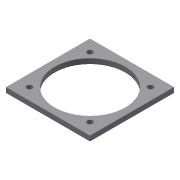
# Autodesk Inventor part: chamberPlateNA11_thin
Saved by Autodesk Inventor 2013 (Build 170138000, 138)
## iProperties
Created: 2012-12-03
Part Number: chamberPlateNA11_thin
Document SubType Name: Modeling
Designer: Ke Si
Density: 1 g/cm^3
Material: Generic
Author: Ke Si
Autodesk Inventor part; units mm, degrees
ref_plane "YZ Plane" through (0, 0, 0) normal (1, 0, 0) x (0, 1, 0)
ref_plane "XZ Plane" through (0, 0, 0) normal (0, 1, 0) x (-1, 0, 0)
ref_plane "XY Plane" through (0, 0, 0) normal (0, 0, 1) x (1, 0, 0)
sketch "Sketch7" plane through (0, 0, 0) normal (0, 1, 0) x (-1, 0, 0)
  line L0 (-25, -25) -> (25, -25)
  line L1 (25, -25) -> (25, 25)
  line L2 (25, 25) -> (-25, 25)
  line L3 (-25, 25) -> (-25, -25)
  line L4 (-25, -25) -> (25, 25) construction
  line L5 (25, -25) -> (-25, 25) construction
  point P0 (0, 0)
  point P1 (0, 0)
  dimension "d54" = 50
  dimension "d55" = 50
  constraints: 12 end point, 2 midpoint
  measures "d54" distance of L2.end L1.end
  measures "d55" distance of L1.end L0.end
extrude "Extrusion4" add sketch "Sketch7" along normal blind 3
sketch "Sketch8" plane through (0, 3, 0) normal (0, 1, 0) x (1, 0, 0)
  circle A0 centre (0, 0) radius 21
  dimension "d58" = 42
  constraints: 1 centre point
  measures "d58" diameter of A0
extrude "Extrusion5" cut sketch "Sketch8" against normal blind 3
sketch "Sketch10" plane through (0, 3, 0) normal (0, 1, 0) x (1, 0, 0)
  line L0 (-18, -18) -> (18, -18)
  line L1 (18, -18) -> (18, 18)
  line L2 (18, 18) -> (-18, 18)
  line L3 (-18, 18) -> (-18, -18)
  line L4 (-18, -18) -> (18, 18) construction
  line L5 (18, -18) -> (-18, 18) construction
  point P0 (0, 0)
  dimension "d62" = 36
  dimension "d63" = 36
  constraints: 12 end point, 2 midpoint
  measures "d62" distance of L2.end L1.end
  measures "d63" distance of L1.end L0.end
hole "Hole2" at (-18, 3, 18) at (-18, 3, -18) at (18, 3, -18) at (18, 3, 18) direction (0, -1, 0) diameter 3.264 end through all clearance for "Flat Head Machine Screw (82)" size "#4" standard "Ansi Unified Screw Threads"
body "Solid3"
